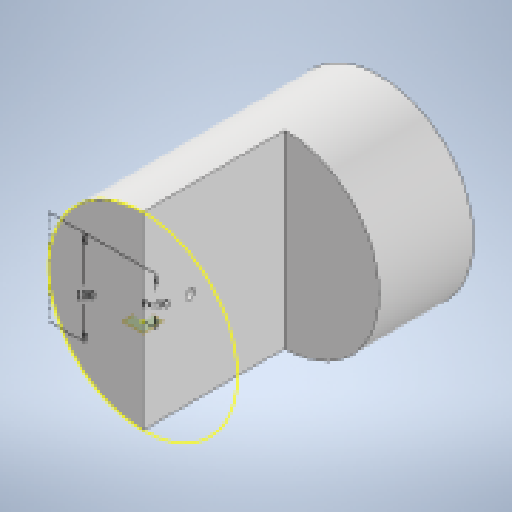
# Autodesk Inventor part: link1
Saved by Autodesk Inventor 2025.4 (Build 294407000, 407)
## iProperties
Created: 2026-03-19
Part Number: link1
Material: Generic
Document SubType Name: Modeling
Designer: dawid
Density: 1 g/cm^3
Appearance: Default
Author: dawid
Autodesk Inventor part; units mm, degrees
ref_plane "YZ Plane" through (0, 0, 0) normal (1, 0, 0) x (0, 1, 0)
ref_plane "XZ Plane" through (0, 0, 0) normal (0, 1, 0) x (-1, 0, 0)
ref_plane "XY Plane" through (0, 0, 0) normal (0, 0, 1) x (1, 0, 0)
sketch "Sketch1" plane through (0, 0, 0) normal (0, 0, 1) x (1, 0, 0)
  circle A0 centre (0, 0) radius 100
  dimension "d0" = 200
  constraints: 1 centre point, 1 coincident
  measures "d0" diameter of A0
extrude "Extrusion1" add sketch "Sketch1" along normal blind 250
sketch "Sketch2" plane through (0, 0, 250) normal (0, 0, 1) x (1, 0, 0)
  circle A0 centre (0, 0) radius 100 projected
  line L0 (-100, 50) -> (-100, -50) construction
  dimension "d3" = 100
  dimension "d4" = 50
  constraints: 2 end point, 1 tangent, 1 vertical
  measures "d3" distance of L0.start L0.end
  measures "d4" vertical distance of point (0, 0) L0.start
ref_plane "Work Plane1" through (0, 0, 250) normal (0, -1, 0) x (1, 0, 0)
sketch "Sketch3" plane through (0, 0, 250) normal (0, -1, 0) x (1, 0, 0)
  line L0 (100, 0) -> (-100, 0) projected
  line L1 (100, 0) -> (0, 0)
  line L2 (0, 0) -> (0, -150)
  line L3 (0, -150) -> (100, -150)
  line L4 (100, -150) -> (100, 0)
  point P0 (0, -250)
  point P1 (0, 0)
  dimension "d6" = 150
  dimension "d17" = 100
  constraints: 8 end point, 2 parallel, 1 horizontal, 1 midpoint, 1 perpendicular
  measures "d6" distance of L1.end L2.end
  measures "d17" distance from line of L1.end L4
extrude "Extrusion2" cut sketch "Sketch3" along normal through all both and the other way through all
sketch "Sketch4" plane through (0, -50, 125) normal (1, 0, 0) x (0, 0, -1)
  circle A0 centre (-75, 50) radius 5
  line L0 (-125, -50) -> (-125, 150) projected
  point P0 (125, 50)
  dimension "d9" = 10
  dimension "d18" = 50
  constraints: 1 centre point
  measures "d9" diameter of A0
  measures "d18" distance from line of L0 A0.centre
hole "Hole1" at (0, 0, 200) direction (-1, 0, 0) diameter 10 end through all
equation "\"d4\" = 0.5 * d3"
equation "\"d18\" = 0.5 * d3"
body "Solid1"
